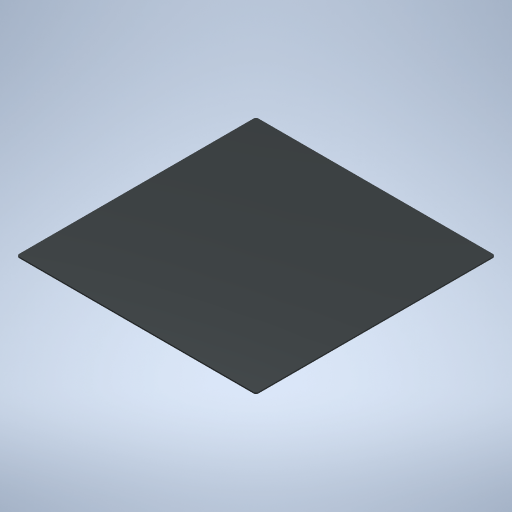
# Autodesk Inventor part: 1mx1m
Saved by Autodesk Inventor 2024.2 (Build 282272000, 272)
## iProperties
Created: 2025-10-02
Part Number: 1mx1m
Material: Hierro, fundido
Document SubType Name: Modeling
Designer: jd.castellanosq
Density: 7.15 g/cm^3
Appearance: Gris hierro
Author: jd.castellanosq
Autodesk Inventor part; units mm, degrees
ref_plane "YZ Plane" through (0, 0, 0) normal (1, 0, 0) x (0, 1, 0)
ref_plane "XZ Plane" through (0, 0, 0) normal (0, 1, 0) x (-1, 0, 0)
ref_plane "XY Plane" through (0, 0, 0) normal (0, 0, 1) x (1, 0, 0)
sketch "Boceto1" plane through (0, 0, 0) normal (0, 0, 1) x (1, 0, 0)
  line L0 (-500, 500) -> (500, 500)
  line L1 (500, 500) -> (500, -500)
  line L2 (500, -500) -> (-500, -500)
  line L3 (-500, -500) -> (-500, 500)
  point P0 (0, 0)
  point P1 (0, 500)
  point P2 (500, 0)
  dimension "d0" = 1000
  constraints: 8 end point, 2 midpoint, 2 parallel, 2 perpendicular, 1 horizontal, 1 horizontal alignment, 1 vertical alignment
  measures "d0" distance of L0.start L0.end
extrude "Extrusión1" add sketch "Boceto1" along normal blind 5
fillet "Empalme1" radius 10 4 edges at (500, 500, 2.5) (-500, 500, 2.5) (500, -500, 2.5) (-500, -500, 2.5)
